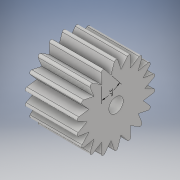
# Autodesk Inventor part: gear
Saved by Autodesk Inventor 2019 (Build 230136000, 136)
## iProperties
Created: 2018-11-15
Part Number: gear
Material: Generic
Document SubType Name: Modeling
Designer: Charlie
Density: 1 g/cm^3
Appearance: Default
Author: Charlie
Autodesk Inventor part; units mm, degrees
ref_plane "YZ Plane" through (0, 0, 0) normal (1, 0, 0) x (0, 1, 0)
ref_plane "XZ Plane" through (0, 0, 0) normal (0, 1, 0) x (-1, 0, 0)
ref_plane "XY Plane" through (0, 0, 0) normal (0, 0, 1) x (1, 0, 0)
sketch "Sketch2" plane through (0, 0, 0) normal (1, 0, 0) x (0, 1, 0)
  circle A0 centre (0, 0) radius 2.54
  line L0 (0, 0) -> (2.54, 0)
  line L1 (0, 0) -> (2.54, 0)
  line L2 (2.54, 0) -> (3.81, 0)
  line L3 (0, 0) -> (2.5014, -0.4411)
  line L4 (0, 0) -> (2.54, 0) construction
  line L5 (2.5014, -0.4411) -> (2.5014, 0.4411)
  line L6 (0, 0) -> (2.5014, 0.4411)
  line L7 (2.5014, 0.4411) -> (3.81, 0)
  line L8 (2.5014, -0.4411) -> (3.81, 0)
  line L9 (2.1997, 1.27) -> (3.5802, 1.3031)
  line L10 (2.3868, 0.8687) -> (3.5802, 1.3031)
  line L11 (2.5014, 0.4411) -> (3.5802, 1.3031)
  line L12 (2.5014, 0.4411) -> (2.1997, 1.27)
  line L13 (0, 0) -> (2.3868, 0.8687)
  line L14 (0, 0) -> (2.1997, 1.27)
  line L15 (0, 0) -> (2.5014, 0.4411)
  line L16 (1.6327, 1.9458) -> (2.9186, 2.449)
  line L17 (1.9458, 1.6327) -> (2.9186, 2.449)
  line L18 (2.1997, 1.27) -> (2.9186, 2.449)
  line L19 (2.1997, 1.27) -> (1.6327, 1.9458)
  line L20 (0, 0) -> (1.9458, 1.6327)
  line L21 (0, 0) -> (1.6327, 1.9458)
  line L22 (0, 0) -> (2.1997, 1.27)
  line L23 (0.8687, 2.3868) -> (1.905, 3.2996)
  line L24 (1.27, 2.1997) -> (1.905, 3.2996)
  line L25 (1.6327, 1.9458) -> (1.905, 3.2996)
  line L26 (1.6327, 1.9458) -> (0.8687, 2.3868)
  line L27 (0, 0) -> (1.27, 2.1997)
  line L28 (0, 0) -> (0.8687, 2.3868)
  line L29 (0, 0) -> (1.6327, 1.9458)
  line L30 (0, 2.54) -> (0.6616, 3.7521)
  line L31 (0.4411, 2.5014) -> (0.6616, 3.7521)
  line L32 (0.8687, 2.3868) -> (0.6616, 3.7521)
  line L33 (0.8687, 2.3868) -> (0, 2.54)
  line L34 (0, 0) -> (0.4411, 2.5014)
  line L35 (0, 0) -> (0, 2.54)
  line L36 (0, 0) -> (0.8687, 2.3868)
  line L37 (-0.8687, 2.3868) -> (-0.6616, 3.7521)
  line L38 (-0.4411, 2.5014) -> (-0.6616, 3.7521)
  line L39 (0, 2.54) -> (-0.6616, 3.7521)
  line L40 (0, 2.54) -> (-0.8687, 2.3868)
  line L41 (0, 0) -> (-0.4411, 2.5014)
  line L42 (0, 0) -> (-0.8687, 2.3868)
  line L43 (0, 0) -> (0, 2.54)
  line L44 (-1.6327, 1.9458) -> (-1.905, 3.2996)
  line L45 (-1.27, 2.1997) -> (-1.905, 3.2996)
  line L46 (-0.8687, 2.3868) -> (-1.905, 3.2996)
  line L47 (-0.8687, 2.3868) -> (-1.6327, 1.9458)
  line L48 (0, 0) -> (-1.27, 2.1997)
  line L49 (0, 0) -> (-1.6327, 1.9458)
  line L50 (0, 0) -> (-0.8687, 2.3868)
  line L51 (-2.1997, 1.27) -> (-2.9186, 2.449)
  line L52 (-1.9458, 1.6327) -> (-2.9186, 2.449)
  line L53 (-1.6327, 1.9458) -> (-2.9186, 2.449)
  line L54 (-1.6327, 1.9458) -> (-2.1997, 1.27)
  line L55 (0, 0) -> (-1.9458, 1.6327)
  line L56 (0, 0) -> (-2.1997, 1.27)
  line L57 (0, 0) -> (-1.6327, 1.9458)
  line L58 (-2.5014, 0.4411) -> (-3.5802, 1.3031)
  line L59 (-2.3868, 0.8687) -> (-3.5802, 1.3031)
  line L60 (-2.1997, 1.27) -> (-3.5802, 1.3031)
  line L61 (-2.1997, 1.27) -> (-2.5014, 0.4411)
  line L62 (0, 0) -> (-2.3868, 0.8687)
  line L63 (0, 0) -> (-2.5014, 0.4411)
  line L64 (0, 0) -> (-2.1997, 1.27)
  line L65 (-2.5014, -0.4411) -> (-3.81, 0)
  line L66 (-2.54, 0) -> (-3.81, 0)
  line L67 (-2.5014, 0.4411) -> (-3.81, 0)
  line L68 (-2.5014, 0.4411) -> (-2.5014, -0.4411)
  line L69 (0, 0) -> (-2.54, 0)
  line L70 (0, 0) -> (-2.5014, -0.4411)
  line L71 (0, 0) -> (-2.5014, 0.4411)
  line L72 (-2.1997, -1.27) -> (-3.5802, -1.3031)
  line L73 (-2.3868, -0.8687) -> (-3.5802, -1.3031)
  line L74 (-2.5014, -0.4411) -> (-3.5802, -1.3031)
  line L75 (-2.5014, -0.4411) -> (-2.1997, -1.27)
  line L76 (0, 0) -> (-2.3868, -0.8687)
  line L77 (0, 0) -> (-2.1997, -1.27)
  line L78 (0, 0) -> (-2.5014, -0.4411)
  line L79 (-1.6327, -1.9458) -> (-2.9186, -2.449)
  line L80 (-1.9458, -1.6327) -> (-2.9186, -2.449)
  line L81 (-2.1997, -1.27) -> (-2.9186, -2.449)
  line L82 (-2.1997, -1.27) -> (-1.6327, -1.9458)
  line L83 (0, 0) -> (-1.9458, -1.6327)
  line L84 (0, 0) -> (-1.6327, -1.9458)
  line L85 (0, 0) -> (-2.1997, -1.27)
  line L86 (-0.8687, -2.3868) -> (-1.905, -3.2996)
  line L87 (-1.27, -2.1997) -> (-1.905, -3.2996)
  line L88 (-1.6327, -1.9458) -> (-1.905, -3.2996)
  line L89 (-1.6327, -1.9458) -> (-0.8687, -2.3868)
  line L90 (0, 0) -> (-1.27, -2.1997)
  line L91 (0, 0) -> (-0.8687, -2.3868)
  line L92 (0, 0) -> (-1.6327, -1.9458)
  line L93 (0, -2.54) -> (-0.6616, -3.7521)
  line L94 (-0.4411, -2.5014) -> (-0.6616, -3.7521)
  line L95 (-0.8687, -2.3868) -> (-0.6616, -3.7521)
  line L96 (-0.8687, -2.3868) -> (0, -2.54)
  line L97 (0, 0) -> (-0.4411, -2.5014)
  line L98 (0, 0) -> (0, -2.54)
  line L99 (0, 0) -> (-0.8687, -2.3868)
  line L100 (0.8687, -2.3868) -> (0.6616, -3.7521)
  line L101 (0.4411, -2.5014) -> (0.6616, -3.7521)
  line L102 (0, -2.54) -> (0.6616, -3.7521)
  line L103 (0, -2.54) -> (0.8687, -2.3868)
  line L104 (0, 0) -> (0.4411, -2.5014)
  line L105 (0, 0) -> (0.8687, -2.3868)
  line L106 (0, 0) -> (0, -2.54)
  line L107 (1.6327, -1.9458) -> (1.905, -3.2996)
  line L108 (1.27, -2.1997) -> (1.905, -3.2996)
  line L109 (0.8687, -2.3868) -> (1.905, -3.2996)
  line L110 (0.8687, -2.3868) -> (1.6327, -1.9458)
  line L111 (0, 0) -> (1.27, -2.1997)
  line L112 (0, 0) -> (1.6327, -1.9458)
  line L113 (0, 0) -> (0.8687, -2.3868)
  line L114 (2.1997, -1.27) -> (2.9186, -2.449)
  line L115 (1.9458, -1.6327) -> (2.9186, -2.449)
  line L116 (1.6327, -1.9458) -> (2.9186, -2.449)
  line L117 (1.6327, -1.9458) -> (2.1997, -1.27)
  line L118 (0, 0) -> (1.9458, -1.6327)
  line L119 (0, 0) -> (2.1997, -1.27)
  line L120 (0, 0) -> (1.6327, -1.9458)
  line L121 (2.5014, -0.4411) -> (3.5802, -1.3031)
  line L122 (2.3868, -0.8687) -> (3.5802, -1.3031)
  line L123 (2.1997, -1.27) -> (3.5802, -1.3031)
  line L124 (2.1997, -1.27) -> (2.5014, -0.4411)
  line L125 (0, 0) -> (2.3868, -0.8687)
  line L126 (0, 0) -> (2.5014, -0.4411)
  line L127 (0, 0) -> (2.1997, -1.27)
  line L128 (2.54, 0) -> (3.302, 0)
  arc A1 (3.4247, -0.1299) -> (3.4255, 0.1291) centre (3.302, 0) ccw
  arc A2 (3.2626, 1.0493) -> (3.1748, 1.2929) centre (3.1029, 1.1294) ccw
  arc A3 (2.707, 2.1019) -> (2.5411, 2.3008) centre (2.5295, 2.1225) ccw
  arc A4 (1.8248, 2.9009) -> (1.601, 3.0311) centre (1.651, 2.8596) ccw
  arc A5 (0.7226, 3.3501) -> (0.4677, 3.3959) centre (0.5734, 3.2518) ccw
  arc A6 (-0.4668, 3.3952) -> (-0.722, 3.3511) centre (-0.5734, 3.2518) ccw
  arc A7 (-1.5999, 3.0308) -> (-1.8246, 2.902) centre (-1.651, 2.8596) ccw
  arc A8 (-2.54, 2.3008) -> (-2.7071, 2.103) centre (-2.5295, 2.1225) ccw
  arc A9 (-3.1738, 1.2934) -> (-3.2631, 1.0503) centre (-3.1029, 1.1294) ccw
  arc A10 (-3.4247, 0.1299) -> (-3.4255, -0.1291) centre (-3.302, 0) ccw
  arc A11 (-3.2626, -1.0493) -> (-3.1748, -1.2929) centre (-3.1029, -1.1294) ccw
  arc A12 (-2.707, -2.1019) -> (-2.5411, -2.3008) centre (-2.5295, -2.1225) ccw
  arc A13 (-1.8248, -2.9009) -> (-1.601, -3.0311) centre (-1.651, -2.8596) ccw
  arc A14 (-0.7226, -3.3501) -> (-0.4677, -3.3959) centre (-0.5734, -3.2518) ccw
  arc A15 (0.4668, -3.3952) -> (0.722, -3.3511) centre (0.5734, -3.2518) ccw
  arc A16 (1.5999, -3.0308) -> (1.8246, -2.902) centre (1.651, -2.8596) ccw
  arc A17 (2.54, -2.3008) -> (2.7071, -2.103) centre (2.5295, -2.1225) ccw
  arc A18 (3.1738, -1.2934) -> (3.2631, -1.0503) centre (3.1029, -1.1294) ccw
  dimension "d3" = 5.08
  dimension "d12" = 1.27
  dimension "d13" = 10
  dimension "d16" = 360
  dimension "d26" = 0.762
  dimension "d27" = 0.259
  dimension "d28" = 43.557
  dimension "d31" = 360
  constraints: 258 end point, 39 point on circle, 19 centre point, 3 horizontal, 2 coincident, 2 point on line, 1 collinear, 1 equal length, 1 vertical, 290 other
  measures "d3" diameter of A0
  measures "d12" distance of L0.end L2.end
  measures "d13" angle of L3 L4
  measures "d26" distance of L4.end L128.end
  measures "d27" distance of A1.start A1.end
extrude "Extrusion1" add sketch "Sketch2" along normal blind 4.572
sketch "Sketch3" plane through (4.572, 0, 0) normal (1, 0, 0) x (0, 0, -1)
  circle A0 centre (0, 0) radius 0.635
  dimension "d20" = 1.27
  constraints: 1 centre point, 1 coincident
  measures "d20" diameter of A0
extrude "Extrusion2" cut sketch "Sketch3" against normal blind 4.572
sketch "Sketch4" plane through (4.572, 0, 0) normal (1, 0, 0) x (0, 0, -1)
  line L0 (0, 0) -> (0, 3.302)
  circle A0 centre (0, 3.302) radius 0.1623
  line L1 (0.4411, 2.5014) -> (0, 3.81) projected
  line L2 (0, 3.81) -> (-0.4411, 2.5014) projected
  line L3 (-0.1538, 3.3538) -> (0, 3.81)
  line L4 (0, 3.81) -> (0.1538, 3.3538)
  arc A1 (0.1538, 3.3538) -> (-0.1538, 3.3538) centre (0, 3.302) ccw
  line L5 (-1.2916, 3.099) -> (-1.3031, 3.5802)
  line L6 (-1.3031, 3.5802) -> (-1.0026, 3.2042)
  arc A2 (-1.0026, 3.2042) -> (-1.2916, 3.099) centre (-1.1294, 3.1029) ccw
  line L7 (-2.2736, 2.4703) -> (-2.449, 2.9186)
  line L8 (-2.449, 2.9186) -> (-2.038, 2.668)
  arc A3 (-2.038, 2.668) -> (-2.2736, 2.4703) centre (-2.1225, 2.5295) ccw
  line L9 (-2.9814, 1.5438) -> (-3.2996, 1.905)
  line L10 (-3.2996, 1.905) -> (-2.8276, 1.8101)
  arc A4 (-2.8276, 1.8101) -> (-2.9814, 1.5438) centre (-2.8596, 1.651) ccw
  line L11 (-3.3296, 0.431) -> (-3.7521, 0.6616)
  line L12 (-3.7521, 0.6616) -> (-3.2762, 0.7338)
  arc A5 (-3.2762, 0.7338) -> (-3.3296, 0.431) centre (-3.2518, 0.5734) ccw
  line L13 (-3.2762, -0.7338) -> (-3.7521, -0.6616)
  line L14 (-3.7521, -0.6616) -> (-3.3296, -0.431)
  arc A6 (-3.3296, -0.431) -> (-3.2762, -0.7338) centre (-3.2518, -0.5734) ccw
  line L15 (-2.8276, -1.8101) -> (-3.2996, -1.905)
  line L16 (-3.2996, -1.905) -> (-2.9814, -1.5438)
  arc A7 (-2.9814, -1.5438) -> (-2.8276, -1.8101) centre (-2.8596, -1.651) ccw
  line L17 (-2.038, -2.668) -> (-2.449, -2.9186)
  line L18 (-2.449, -2.9186) -> (-2.2736, -2.4703)
  arc A8 (-2.2736, -2.4703) -> (-2.038, -2.668) centre (-2.1225, -2.5295) ccw
  line L19 (-1.0026, -3.2042) -> (-1.3031, -3.5802)
  line L20 (-1.3031, -3.5802) -> (-1.2916, -3.099)
  arc A9 (-1.2916, -3.099) -> (-1.0026, -3.2042) centre (-1.1294, -3.1029) ccw
  line L21 (0.1538, -3.3538) -> (0, -3.81)
  line L22 (0, -3.81) -> (-0.1538, -3.3538)
  arc A10 (-0.1538, -3.3538) -> (0.1538, -3.3538) centre (0, -3.302) ccw
  line L23 (1.2916, -3.099) -> (1.3031, -3.5802)
  line L24 (1.3031, -3.5802) -> (1.0026, -3.2042)
  arc A11 (1.0026, -3.2042) -> (1.2916, -3.099) centre (1.1294, -3.1029) ccw
  line L25 (2.2736, -2.4703) -> (2.449, -2.9186)
  line L26 (2.449, -2.9186) -> (2.038, -2.668)
  arc A12 (2.038, -2.668) -> (2.2736, -2.4703) centre (2.1225, -2.5295) ccw
  line L27 (2.9814, -1.5438) -> (3.2996, -1.905)
  line L28 (3.2996, -1.905) -> (2.8276, -1.8101)
  arc A13 (2.8276, -1.8101) -> (2.9814, -1.5438) centre (2.8596, -1.651) ccw
  line L29 (3.3296, -0.431) -> (3.7521, -0.6616)
  line L30 (3.7521, -0.6616) -> (3.2762, -0.7338)
  arc A14 (3.2762, -0.7338) -> (3.3296, -0.431) centre (3.2518, -0.5734) ccw
  line L31 (3.2762, 0.7338) -> (3.7521, 0.6616)
  line L32 (3.7521, 0.6616) -> (3.3296, 0.431)
  arc A15 (3.3296, 0.431) -> (3.2762, 0.7338) centre (3.2518, 0.5734) ccw
  line L33 (2.8276, 1.8101) -> (3.2996, 1.905)
  line L34 (3.2996, 1.905) -> (2.9814, 1.5438)
  arc A16 (2.9814, 1.5438) -> (2.8276, 1.8101) centre (2.8596, 1.651) ccw
  line L35 (2.038, 2.668) -> (2.449, 2.9186)
  line L36 (2.449, 2.9186) -> (2.2736, 2.4703)
  arc A17 (2.2736, 2.4703) -> (2.038, 2.668) centre (2.1225, 2.5295) ccw
  line L37 (1.0026, 3.2042) -> (1.3031, 3.5802)
  line L38 (1.3031, 3.5802) -> (1.2916, 3.099)
  arc A18 (1.2916, 3.099) -> (1.0026, 3.2042) centre (1.1294, 3.1029) ccw
  dimension "d33" = 3.302
  dimension "d36" = 360
  constraints: 74 end point, 38 point on circle, 19 centre point, 2 coincident, 2 point on line, 1 collinear, 1 tangent, 1 vertical, 127 other
  measures "d33" distance of L0.start L0.end
extrude "Extrusion3" cut sketch "Sketch4" against normal blind 4.572 contours A0 L2 L1 | L5 L6 A2 | L7 L8 A3 | L9 L10 A4 | L11 L12 A5 | L13 L14 A6 | L15 L16 A7 | L17 L18 A8 | L19 L20 A9 | L21 L22 A10 | L23 L24 A11 | L25 L26 A12 | L27 L28 A13 | L29 L30 A14 | L31 L32 A15 | L33 L34 A16 | L35 L36 A17 | L37 L38 A18
body "Solid1"
